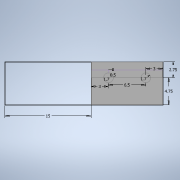
# Autodesk Inventor part: limit switch mount
Saved by Autodesk Inventor 2022 (Build 260153000, 153)
## iProperties
Created: 2022-02-19
Part Number: limit switch mount
Material: Generic
Document SubType Name: Modeling
Designer: a-dubs
Density: 1 g/cm^3
Appearance: Default
Author: a-dubs
Autodesk Inventor part; units mm, degrees
ref_plane "YZ Plane" through (0, 0, 0) normal (1, 0, 0) x (0, 1, 0)
ref_plane "XZ Plane" through (0, 0, 0) normal (0, 1, 0) x (-1, 0, 0)
ref_plane "XY Plane" through (0, 0, 0) normal (0, 0, 1) x (1, 0, 0)
sketch "Sketch1" plane through (0, 0, 0) normal (0, 0, 1) x (1, 0, 0)
  line L0 (0, 0) -> (6.5, 0)
  circle A0 centre (0, 0) radius 0.85
  circle A1 centre (6.5, 0) radius 0.85
  line L1 (0, 0) -> (-3, 0)
  line L2 (6.5, 0) -> (9.5, 0)
  line L3 (-3, 0) -> (-3, 4.75)
  line L4 (9.5, 0) -> (9.5, 4.75)
  line L5 (-3, 0) -> (-3, -2.75)
  line L6 (9.5, 0) -> (9.5, -2.75)
  line L7 (9.5, -2.75) -> (-3, -2.75)
  line L8 (-3, 4.75) -> (9.5, 4.75)
  line L9 (9.5, 4.75) -> (24.5, 4.75)
  line L10 (9.5, -2.75) -> (24.5, -2.75)
  line L11 (24.5, -2.75) -> (24.5, 4.75)
  line L12 (6.5, -0.85) -> (6.5, -1.35)
  line L13 (6.5, -1.35) -> (9.5, -1.35)
  line L14 (9.5, -1.35) -> (9.5, -2.75)
  line L15 (6.5, -1.35) -> (-3, -1.35)
  dimension "d2" = 1.7
  dimension "d0" = 6.5
  dimension "d1" = 1.7
  dimension "d3" = 3
  dimension "d4" = 3
  dimension "d5" = 4.75
  dimension "d6" = 2.75
  dimension "d9" = 15
  dimension "d10" = 0.5
  constraints: 32 end point, 6 horizontal, 4 perpendicular, 4 vertical, 2 coincident, 2 parallel, 2 point on line, 1 centre point, 1 collinear, 1 vertical alignment, 2 other
  measures "d0" distance of L0.start L0.end
  measures "d1" diameter of A0
  measures "d3" distance of L1.start L1.end
  measures "d4" distance of L2.start L2.end
  measures "d5" distance of L1.end L3.end
  measures "d6" distance of L1.end L5.end
  measures "d9" distance of L4.end L9.end
  measures "d10" distance of L12.start L12.end
extrude "Extrusion1" add sketch "Sketch1" along normal blind 4 contours L1 A0 L0 | L0 A0 L1 | A0 L1 L3 L8 L4 L2 A1 L0 | L0 A1 L12 L15 L5 L1 A0 | A1 L2 L0 | L0 L2 A1 | L2 L6 L13 L12 A1 | L15 L13 L6 L7 L5
extrude "Extrusion2" add sketch "Sketch1" along normal blind 2.75 from surface at 4 contours L15 L13 L6 L7 L5
extrude "Extrusion3" add sketch "Sketch1" along normal blind 0.3 from surface at 4 contours L1 A0 L0 | L0 A0 L1 | A1 L2 L0 | L0 L2 A1
fillet "Fillet1" radius 0.85 2 edges at (-0.85, 0, 4.3) (5.65, 0, 4.3)
mirror "Mirror1" about plane through (3.25, -2.05, 6.75) normal (0, 0, 1) of "Extrusion3", "Fillet1", "Extrusion2", "Extrusion1"
sketch "Sketch2" plane through (-3, -1.35, 4) normal (0, 1, 0) x (1, 0, 0)
  line L0 (0, 0) -> (0, -5.5) projected
  line L1 (0, 0) -> (0, -5.5)
  line L2 (12.5, -5.5) -> (0, -5.5) projected
  line L3 (0, -5.5) -> (12.5, -5.5)
  line L4 (12.5, 0) -> (12.5, -5.5) projected
  line L5 (12.5, -5.5) -> (12.5, 0)
  line L6 (12.5, 0) -> (0, 0)
  line L7 (0, -2.75) -> (12.5, -2.75)
  line L8 (0, -2.75) -> (1.8, -2.75)
  line L9 (12.5, -2.75) -> (0.7, -2.75)
  line L10 (12.5, -2.75) -> (10.7, -2.75)
  line L11 (0, -2.75) -> (11.8, -2.75)
  line L12 (6.25, -2.75) -> (5.7, -2.75)
  line L13 (6.25, -2.75) -> (6.8, -2.75)
  line L14 (0, -2.75) -> (0, -2.45)
  line L15 (0, -2.75) -> (0, -3.05)
  line L16 (0, -3.05) -> (12.5, -3.05)
  line L17 (12.5, -2.45) -> (0, -2.45)
  line L18 (0.7, -2.45) -> (0.7, -3.05)
  line L19 (1.8, -2.45) -> (1.8, -3.05)
  line L20 (5.7, -2.45) -> (5.7, -3.05)
  line L21 (6.8, -3.05) -> (6.8, -2.45)
  line L22 (10.7, -2.45) -> (10.7, -3.05)
  line L23 (11.8, -2.45) -> (11.8, -3.05)
  point P0 (3, 4)
  dimension "d16" = 1.8
  dimension "d17" = 11.8
  dimension "d18" = 1.8
  dimension "d19" = 11.8
  dimension "d20" = 0.55
  dimension "d21" = 0.55
  dimension "d22" = 0.3
  dimension "d23" = 0.3
  constraints: 42 end point, 23 point on line, 8 perpendicular, 4 equal length, 2 midpoint
  measures "d16" distance of L7.start L8.end
  measures "d17" distance of L7.end L9.end
  measures "d18" distance of L7.end L10.end
  measures "d19" distance of L7.start L11.end
  measures "d20" distance of L12.start L12.end
  measures "d21" distance of L12.start L13.end
  measures "d22" distance of L7.start L14.end
  measures "d23" distance of L7.start L15.end
extrude "Extrusion4" [suppressed]
extrude "Extrusion5" [suppressed]
extrude "Extrusion6" [suppressed]
extrude "Extrusion7" [suppressed]
sketch "Sketch3" plane through (-3, 4.75, 4) normal (0, 1, 0) x (1, 0, 0)
  line L0 (12.5, 4) -> (0, 4) projected
  line L1 (0, -9.5) -> (12.5, -9.5) projected
  line L2 (12.5, 4) -> (12.5, -9.5)
  line L3 (12.5, 0) -> (12.5, -5.5) projected
  line L4 (12.5, -2.75) -> (27.5, -2.75)
  line L5 (27.5, -14.5) -> (27.5, 9) projected
  line L6 (12.5, -2.75) -> (13, -2.75)
  line L7 (13, -2.75) -> (16.2, -2.75)
  line L8 (16.2, -2.75) -> (16.2, 6.8335)
  circle A0 centre (16.2, 6.8335) radius 1.6
  line L9 (16.2, -2.75) -> (16.2, -12.3335)
  circle A1 centre (16.2, -12.3335) radius 1.6
  circle A2 centre (22.6, 6.8335) radius 1.6
  line L10 (22.6, -2.75) -> (22.6, 6.8335)
  line L11 (22.6, -2.75) -> (22.6, -12.3335)
  circle A3 centre (22.6, -12.3335) radius 1.6
  point P0 (3, 4)
  dimension "d32" = 0.5
  dimension "d33" = 3.2
  dimension "d34" = 9.5835
  dimension "d35" = 3.2
  dimension "d38" = 6.4
  constraints: 16 end point, 4 centre point, 4 coincident, 2 midpoint, 2 point on line, 2 symmetric about line, 2 vertical, 1 horizontal, 10 other
  measures "d32" distance of L4.start L6.end
  measures "d33" distance of L6.end L7.end
  measures "d34" distance of L7.end L8.end
  measures "d35" diameter of A0
  measures "d38" distance of A0.centre A2.centre
extrude "Extrusion8" [suppressed]
equation "\"d15\" = 0.5 * d1"
body "Solid1"
